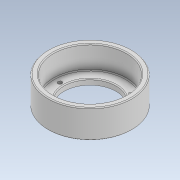
# Autodesk Inventor part: front_hip_mask
Saved by Autodesk Inventor 2020 (Build 240168000, 168)
## iProperties
Created: 2021-02-08
Part Number: front_hip_mask
Material: Generic
Document SubType Name: Modeling
Designer: DELL
Density: 1 g/cm^3
Appearance: Default
Author: DELL
Autodesk Inventor part; units mm, degrees
ref_plane "YZ Plane" through (0, 0, 0) normal (1, 0, 0) x (0, 1, 0)
ref_plane "XZ Plane" through (0, 0, 0) normal (0, 1, 0) x (-1, 0, 0)
ref_plane "XY Plane" through (0, 0, 0) normal (0, 0, 1) x (1, 0, 0)
sketch "Sketch1" plane through (0, 0, 0) normal (0, 1, 0) x (-1, 0, 0)
  circle A0 centre (0, 0) radius 46
  circle A1 centre (0, 0) radius 40
  circle A2 centre (0, 0) radius 28.5
  circle A3 centre (0, 0) radius 33 construction
  line L0 (0, 0) -> (16.5, 28.5788) construction
  line L1 (46, 0) -> (-46, 0) construction
  circle A4 centre (33, 0) radius 2.25
  circle A5 centre (16.5, 28.5788) radius 2.25
  circle A6 centre (33, 0) radius 3.75
  circle A7 centre (16.5, 28.5788) radius 3.75
  line L2 (0, 46) -> (0, -46) construction
  circle A8 centre (16.5, -28.5788) radius 2.25
  circle A9 centre (16.5, -28.5788) radius 3.75
  circle A10 centre (-16.5, 28.5788) radius 2.25
  circle A11 centre (-16.5, 28.5788) radius 3.75
  circle A12 centre (-16.5, -28.5788) radius 3.75
  circle A13 centre (-16.5, -28.5788) radius 2.25
  line L3 (0, 0) -> (-16.5, 28.5788) construction
  line L4 (-20, 34.641) -> (-0.3277, 45.9988)
  line L5 (-16.5, 28.5788) -> (-20, 34.641) construction
  line L6 (-20, -34.641) -> (-0.3277, -45.9988)
  dimension "d0" = 92
  dimension "d1" = 80
  dimension "d2" = 57
  dimension "d3" = 66
  dimension "d4" = 60
  dimension "d5" = 4.5
  dimension "d6" = 7.5
  constraints: 14 centre point, 14 end point, 10 coincident, 9 point on circle, 8 symmetric about line, 3 midpoint, 2 equal radius, 2 point on line, 1 collinear, 1 horizontal, 1 tangent, 1 vertical, 6 other
  measures "d0" diameter of A0
  measures "d1" diameter of A1
  measures "d2" diameter of A2
  measures "d3" diameter of A3
  measures "d4" angle of L1 L0
  measures "d5" diameter of A4
  measures "d6" diameter of A6
extrude "Extrusion1" add sketch "Sketch1" along normal blind 6 contours A0 L6 A1 L4 | L4 A1 L6 A0 | A1 | A5 | A6 | A7 | A8 | A9 | A11 | A12
extrude "Extrusion2" add sketch "Sketch1" along normal blind 25 from surface at 6 contours A0 L6 A1 L4 | L4 A1 L6 A0
fillet "Fillet1" [suppressed]
fillet "Fillet2" [suppressed]
fillet "Fillet3" radius 1 5 edges at (-20, 6, 34.641) (-0.3277, 31, -45.9988) (-20, 31, 34.641) (-0.3277, 0, -45.9988) (28.5, 6, 0)
extrude "Extrusion3" cut sketch "Sketch1" along normal blind 3 contours A4 | A6 | A10 | A11 | A12 | A13
body "Solid1"
